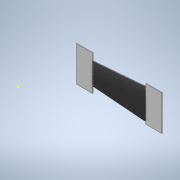
# Autodesk Inventor part: Device21
Saved by Autodesk Inventor 2020 (Build 240168000, 168)
## iProperties
Created: 2020-05-14
Part Number: Device21
Material: Generic
Document SubType Name: Modeling
Designer: nicva
Density: 1 g/cm^3
Appearance: Default
Autodesk Inventor part; units mm, degrees
ref_plane "YZ Plane" through (0, 0, 0) normal (1, 0, 0) x (0, 1, 0)
ref_plane "XZ Plane" through (0, 0, 0) normal (0, 1, 0) x (-1, 0, 0)
ref_plane "XY Plane" through (0, 0, 0) normal (0, 0, 1) x (1, 0, 0)
sketch "Sketch1" plane through (0, 0, 0) normal (0, 0, 1) x (1, 0, 0)
  point P0 (0, 0)
sketch "0" plane through (0, 0, 0) normal (0, 0, 1) x (1, 0, 0)
  line L0 (23.8209, 9.2756) -> (23.8209, 9.3229)
  line L1 (14.0209, 9.269) -> (23.8209, 9.2756)
  line L2 (14.0209, 9.303) -> (23.8209, 9.3229)
  line L3 (23.8209, 9.4649) -> (23.8209, 9.5122)
  line L4 (14.0209, 9.4049) -> (23.8209, 9.4649)
  line L5 (14.0209, 9.4389) -> (23.8209, 9.5122)
  line L6 (23.8209, 9.6542) -> (23.8209, 9.7015)
  line L7 (14.0209, 9.5409) -> (23.8209, 9.6542)
  line L8 (14.0209, 9.5749) -> (23.8209, 9.7015)
  line L9 (23.8209, 9.8435) -> (23.8209, 9.8908)
  line L10 (14.0209, 9.6769) -> (23.8209, 9.8435)
  line L11 (14.0209, 9.7109) -> (23.8209, 9.8908)
  line L12 (23.8209, 10.0328) -> (23.8209, 10.0801)
  line L13 (14.0209, 9.8129) -> (23.8209, 10.0328)
  line L14 (14.0209, 9.8469) -> (23.8209, 10.0801)
  line L15 (23.8209, 10.2221) -> (23.8209, 10.2694)
  line L16 (14.0209, 9.9489) -> (23.8209, 10.2221)
  line L17 (14.0209, 9.9829) -> (23.8209, 10.2694)
  line L18 (23.8209, 10.4113) -> (23.8209, 10.4587)
  line L19 (14.0209, 10.0848) -> (23.8209, 10.4113)
  line L20 (14.0209, 10.1188) -> (23.8209, 10.4587)
  line L21 (23.8209, 10.6006) -> (23.8209, 10.6479)
  line L22 (14.0209, 10.2208) -> (23.8209, 10.6006)
  line L23 (14.0209, 10.2548) -> (23.8209, 10.6479)
  line L24 (23.8209, 10.7899) -> (23.8209, 10.8372)
  line L25 (14.0209, 10.3568) -> (23.8209, 10.7899)
  line L26 (14.0209, 10.3908) -> (23.8209, 10.8372)
  line L27 (23.8209, 10.9792) -> (23.8209, 11.0265)
  line L28 (14.0209, 10.4928) -> (23.8209, 10.9792)
  line L29 (14.0209, 10.5268) -> (23.8209, 11.0265)
  line L30 (23.8209, 11.1685) -> (23.8209, 11.2158)
  line L31 (14.0209, 10.6288) -> (23.8209, 11.1685)
  line L32 (14.0209, 10.6628) -> (23.8209, 11.2158)
  line L33 (23.8209, 11.3578) -> (23.8209, 11.4051)
  line L34 (14.0209, 10.7648) -> (23.8209, 11.3578)
  line L35 (14.0209, 10.7988) -> (23.8209, 11.4051)
  line L36 (23.8209, 11.5471) -> (23.8209, 11.5944)
  line L37 (14.0209, 10.9007) -> (23.8209, 11.5471)
  line L38 (14.0209, 10.9347) -> (23.8209, 11.5944)
  line L39 (23.8209, 11.7363) -> (23.8209, 11.7837)
  line L40 (14.0209, 11.0367) -> (23.8209, 11.7363)
  line L41 (14.0209, 11.0707) -> (23.8209, 11.7837)
  line L42 (23.8209, 11.9256) -> (23.8209, 11.9729)
  line L43 (14.0209, 11.1727) -> (23.8209, 11.9256)
  line L44 (14.0209, 11.2067) -> (23.8209, 11.9729)
  line L45 (14.0209, 9.303) -> (14.0209, 9.4049)
  line L46 (14.0209, 9.4389) -> (14.0209, 9.5409)
  line L47 (14.0209, 9.5749) -> (14.0209, 9.6769)
  line L48 (14.0209, 9.7109) -> (14.0209, 9.8129)
  line L49 (14.0209, 9.8469) -> (14.0209, 9.9489)
  line L50 (14.0209, 9.9829) -> (14.0209, 10.0848)
  line L51 (14.0209, 10.1188) -> (14.0209, 10.2208)
  line L52 (14.0209, 10.2548) -> (14.0209, 10.3568)
  line L53 (14.0209, 10.3908) -> (14.0209, 10.4928)
  line L54 (14.0209, 10.5268) -> (14.0209, 10.6288)
  line L55 (14.0209, 10.6628) -> (14.0209, 10.7648)
  line L56 (14.0209, 10.7988) -> (14.0209, 10.9007)
  line L57 (14.0209, 10.9347) -> (14.0209, 11.0367)
  line L58 (14.0209, 11.0707) -> (14.0209, 11.1727)
  line L59 (23.8209, 9.0863) -> (23.8209, 9.1337)
  line L60 (14.0209, 9.133) -> (23.8209, 9.0863)
  line L61 (14.0209, 9.167) -> (23.8209, 9.1337)
  line L62 (23.8209, 8.8971) -> (23.8209, 8.9444)
  line L63 (14.0209, 8.997) -> (23.8209, 8.8971)
  line L64 (14.0209, 9.031) -> (23.8209, 8.9444)
  line L65 (23.8209, 8.7078) -> (23.8209, 8.7551)
  line L66 (14.0209, 8.861) -> (23.8209, 8.7078)
  line L67 (14.0209, 8.895) -> (23.8209, 8.7551)
  line L68 (23.8209, 8.5185) -> (23.8209, 8.5658)
  line L69 (14.0209, 8.725) -> (23.8209, 8.5185)
  line L70 (14.0209, 8.759) -> (23.8209, 8.5658)
  line L71 (23.8209, 8.3292) -> (23.8209, 8.3765)
  line L72 (14.0209, 8.5891) -> (23.8209, 8.3292)
  line L73 (14.0209, 8.6231) -> (23.8209, 8.3765)
  line L74 (23.8209, 8.1399) -> (23.8209, 8.1872)
  line L75 (14.0209, 8.4531) -> (23.8209, 8.1399)
  line L76 (14.0209, 8.4871) -> (23.8209, 8.1872)
  line L77 (23.8209, 7.9506) -> (23.8209, 7.9979)
  line L78 (14.0209, 8.3171) -> (23.8209, 7.9506)
  line L79 (14.0209, 8.3511) -> (23.8209, 7.9979)
  line L80 (23.8209, 7.7613) -> (23.8209, 7.8087)
  line L81 (14.0209, 8.1811) -> (23.8209, 7.7613)
  line L82 (14.0209, 8.2151) -> (23.8209, 7.8087)
  line L83 (23.8209, 7.5721) -> (23.8209, 7.6194)
  line L84 (14.0209, 8.0451) -> (23.8209, 7.5721)
  line L85 (14.0209, 8.0791) -> (23.8209, 7.6194)
  line L86 (23.8209, 7.3828) -> (23.8209, 7.4301)
  line L87 (14.0209, 7.9092) -> (23.8209, 7.3828)
  line L88 (14.0209, 7.9431) -> (23.8209, 7.4301)
  line L89 (23.8209, 7.1935) -> (23.8209, 7.2408)
  line L90 (14.0209, 7.7732) -> (23.8209, 7.1935)
  line L91 (14.0209, 7.8072) -> (23.8209, 7.2408)
  line L92 (23.8209, 7.0042) -> (23.8209, 7.0515)
  line L93 (14.0209, 7.6372) -> (23.8209, 7.0042)
  line L94 (14.0209, 7.6712) -> (23.8209, 7.0515)
  line L95 (23.8209, 6.8149) -> (23.8209, 6.8622)
  line L96 (14.0209, 7.5012) -> (23.8209, 6.8149)
  line L97 (14.0209, 7.5352) -> (23.8209, 6.8622)
  line L98 (23.8209, 6.6256) -> (23.8209, 6.6729)
  line L99 (14.0209, 7.3652) -> (23.8209, 6.6256)
  line L100 (14.0209, 7.3992) -> (23.8209, 6.6729)
  line L101 (23.8209, 6.4363) -> (23.8209, 6.4837)
  line L102 (14.0209, 7.2292) -> (23.8209, 6.4363)
  line L103 (14.0209, 7.2632) -> (23.8209, 6.4837)
  line L104 (14.0209, 9.133) -> (14.0209, 9.031)
  line L105 (14.0209, 8.997) -> (14.0209, 8.895)
  line L106 (14.0209, 8.861) -> (14.0209, 8.759)
  line L107 (14.0209, 8.725) -> (14.0209, 8.6231)
  line L108 (14.0209, 8.5891) -> (14.0209, 8.4871)
  line L109 (14.0209, 8.4531) -> (14.0209, 8.3511)
  line L110 (14.0209, 8.3171) -> (14.0209, 8.2151)
  line L111 (14.0209, 8.1811) -> (14.0209, 8.0791)
  line L112 (14.0209, 8.0451) -> (14.0209, 7.9431)
  line L113 (14.0209, 7.9092) -> (14.0209, 7.8072)
  line L114 (14.0209, 7.7732) -> (14.0209, 7.6712)
  line L115 (14.0209, 7.6372) -> (14.0209, 7.5352)
  line L116 (14.0209, 7.5012) -> (14.0209, 7.3992)
  line L117 (14.0209, 7.3652) -> (14.0209, 7.2632)
  line L118 (14.0209, 9.167) -> (14.0209, 9.269)
  line L119 (14.2209, 9.3376) -> (14.2209, 9.3719)
  line L120 (14.2209, 9.3376) -> (24.0209, 9.3709)
  line L121 (14.2209, 9.3719) -> (24.0209, 9.4185)
  line L122 (14.2209, 9.4747) -> (14.2209, 9.509)
  line L123 (14.2209, 9.4747) -> (24.0209, 9.5613)
  line L124 (14.2209, 9.509) -> (24.0209, 9.6089)
  line L125 (14.2209, 9.6118) -> (14.2209, 9.646)
  line L126 (14.2209, 9.6118) -> (24.0209, 9.7517)
  line L127 (14.2209, 9.646) -> (24.0209, 9.7993)
  line L128 (14.2209, 9.7488) -> (14.2209, 9.7831)
  line L129 (14.2209, 9.7488) -> (24.0209, 9.9421)
  line L130 (14.2209, 9.7831) -> (24.0209, 9.9897)
  line L131 (14.2209, 9.8859) -> (14.2209, 9.9202)
  line L132 (14.2209, 9.8859) -> (24.0209, 10.1324)
  line L133 (14.2209, 9.9202) -> (24.0209, 10.18)
  line L134 (14.2209, 10.023) -> (14.2209, 10.0572)
  line L135 (14.2209, 10.023) -> (24.0209, 10.3228)
  line L136 (14.2209, 10.0572) -> (24.0209, 10.3704)
  line L137 (14.2209, 10.16) -> (14.2209, 10.1943)
  line L138 (14.2209, 10.16) -> (24.0209, 10.5132)
  line L139 (14.2209, 10.1943) -> (24.0209, 10.5608)
  line L140 (14.2209, 10.2971) -> (14.2209, 10.3314)
  line L141 (14.2209, 10.2971) -> (24.0209, 10.7036)
  line L142 (14.2209, 10.3314) -> (24.0209, 10.7512)
  line L143 (14.2209, 10.4342) -> (14.2209, 10.4685)
  line L144 (14.2209, 10.4342) -> (24.0209, 10.8939)
  line L145 (14.2209, 10.4685) -> (24.0209, 10.9415)
  line L146 (14.2209, 10.5713) -> (14.2209, 10.6055)
  line L147 (14.2209, 10.5713) -> (24.0209, 11.0843)
  line L148 (14.2209, 10.6055) -> (24.0209, 11.1319)
  line L149 (14.2209, 10.7083) -> (14.2209, 10.7426)
  line L150 (14.2209, 10.7083) -> (24.0209, 11.2747)
  line L151 (14.2209, 10.7426) -> (24.0209, 11.3223)
  line L152 (14.2209, 10.8454) -> (14.2209, 10.8797)
  line L153 (14.2209, 10.8454) -> (24.0209, 11.4651)
  line L154 (14.2209, 10.8797) -> (24.0209, 11.5127)
  line L155 (14.2209, 10.9825) -> (14.2209, 11.0167)
  line L156 (14.2209, 10.9825) -> (24.0209, 11.6554)
  line L157 (14.2209, 11.0167) -> (24.0209, 11.703)
  line L158 (14.2209, 11.1195) -> (14.2209, 11.1538)
  line L159 (14.2209, 11.1195) -> (24.0209, 11.8458)
  line L160 (14.2209, 11.1538) -> (24.0209, 11.8934)
  line L161 (14.2209, 11.2566) -> (14.2209, 11.2909)
  line L162 (14.2209, 11.2566) -> (24.0209, 12.0362)
  line L163 (14.2209, 11.2909) -> (24.0209, 12.0838)
  line L164 (24.0209, 9.4185) -> (24.0209, 9.5613)
  line L165 (24.0209, 9.6089) -> (24.0209, 9.7517)
  line L166 (24.0209, 9.7993) -> (24.0209, 9.9421)
  line L167 (24.0209, 9.9897) -> (24.0209, 10.1324)
  line L168 (24.0209, 10.18) -> (24.0209, 10.3228)
  line L169 (24.0209, 10.3704) -> (24.0209, 10.5132)
  line L170 (24.0209, 10.5608) -> (24.0209, 10.7036)
  line L171 (24.0209, 10.7512) -> (24.0209, 10.8939)
  line L172 (24.0209, 10.9415) -> (24.0209, 11.0843)
  line L173 (24.0209, 11.1319) -> (24.0209, 11.2747)
  line L174 (24.0209, 11.3223) -> (24.0209, 11.4651)
  line L175 (24.0209, 11.5127) -> (24.0209, 11.6554)
  line L176 (24.0209, 11.703) -> (24.0209, 11.8458)
  line L177 (24.0209, 11.8934) -> (24.0209, 12.0362)
  line L178 (14.2209, 9.2006) -> (14.2209, 9.2348)
  line L179 (14.2209, 9.2006) -> (24.0209, 9.1806)
  line L180 (14.2209, 9.2348) -> (24.0209, 9.2282)
  line L181 (14.2209, 9.0635) -> (14.2209, 9.0978)
  line L182 (14.2209, 9.0635) -> (24.0209, 8.9902)
  line L183 (14.2209, 9.0978) -> (24.0209, 9.0378)
  line L184 (14.2209, 8.9264) -> (14.2209, 8.9607)
  line L185 (14.2209, 8.9264) -> (24.0209, 8.7998)
  line L186 (14.2209, 8.9607) -> (24.0209, 8.8474)
  line L187 (14.2209, 8.7894) -> (14.2209, 8.8236)
  line L188 (14.2209, 8.7894) -> (24.0209, 8.6095)
  line L189 (14.2209, 8.8236) -> (24.0209, 8.657)
  line L190 (14.2209, 8.6523) -> (14.2209, 8.6866)
  line L191 (14.2209, 8.6523) -> (24.0209, 8.4191)
  line L192 (14.2209, 8.6866) -> (24.0209, 8.4667)
  line L193 (14.2209, 8.5152) -> (14.2209, 8.5495)
  line L194 (14.2209, 8.5152) -> (24.0209, 8.2287)
  line L195 (14.2209, 8.5495) -> (24.0209, 8.2763)
  line L196 (14.2209, 8.3782) -> (14.2209, 8.4124)
  line L197 (14.2209, 8.3782) -> (24.0209, 8.0383)
  line L198 (14.2209, 8.4124) -> (24.0209, 8.0859)
  line L199 (14.2209, 8.2411) -> (14.2209, 8.2753)
  line L200 (14.2209, 8.2411) -> (24.0209, 7.848)
  line L201 (14.2209, 8.2753) -> (24.0209, 7.8956)
  line L202 (14.2209, 8.104) -> (14.2209, 8.1383)
  line L203 (14.2209, 8.104) -> (24.0209, 7.6576)
  line L204 (14.2209, 8.1383) -> (24.0209, 7.7052)
  line L205 (14.2209, 7.9669) -> (14.2209, 8.0012)
  line L206 (14.2209, 7.9669) -> (24.0209, 7.4672)
  line L207 (14.2209, 8.0012) -> (24.0209, 7.5148)
  line L208 (14.2209, 7.8299) -> (14.2209, 7.8641)
  line L209 (14.2209, 7.8299) -> (24.0209, 7.2768)
  line L210 (14.2209, 7.8641) -> (24.0209, 7.3244)
  line L211 (14.2209, 7.6928) -> (14.2209, 7.7271)
  line L212 (14.2209, 7.6928) -> (24.0209, 7.0865)
  line L213 (14.2209, 7.7271) -> (24.0209, 7.1341)
  line L214 (14.2209, 7.5557) -> (14.2209, 7.59)
  line L215 (14.2209, 7.5557) -> (24.0209, 6.8961)
  line L216 (14.2209, 7.59) -> (24.0209, 6.9437)
  line L217 (14.2209, 7.4187) -> (14.2209, 7.4529)
  line L218 (14.2209, 7.4187) -> (24.0209, 6.7057)
  line L219 (14.2209, 7.4529) -> (24.0209, 6.7533)
  line L220 (14.2209, 7.2816) -> (14.2209, 7.3159)
  line L221 (14.2209, 7.2816) -> (24.0209, 6.5153)
  line L222 (14.2209, 7.3159) -> (24.0209, 6.5629)
  line L223 (24.0209, 9.1806) -> (24.0209, 9.0378)
  line L224 (24.0209, 8.9902) -> (24.0209, 8.8474)
  line L225 (24.0209, 8.7998) -> (24.0209, 8.657)
  line L226 (24.0209, 8.6095) -> (24.0209, 8.4667)
  line L227 (24.0209, 8.4191) -> (24.0209, 8.2763)
  line L228 (24.0209, 8.2287) -> (24.0209, 8.0859)
  line L229 (24.0209, 8.0383) -> (24.0209, 7.8956)
  line L230 (24.0209, 7.848) -> (24.0209, 7.7052)
  line L231 (24.0209, 7.6576) -> (24.0209, 7.5148)
  line L232 (24.0209, 7.4672) -> (24.0209, 7.3244)
  line L233 (24.0209, 7.2768) -> (24.0209, 7.1341)
  line L234 (24.0209, 7.0865) -> (24.0209, 6.9437)
  line L235 (24.0209, 6.8961) -> (24.0209, 6.7533)
  line L236 (24.0209, 6.7057) -> (24.0209, 6.5629)
  line L237 (24.0209, 9.2282) -> (24.0209, 9.3709)
  line L238 (24.0209, 6.5153) -> (24.0209, 6.0153)
  line L239 (24.0209, 12.0838) -> (24.0209, 12.5838)
  line L240 (24.0209, 6.0153) -> (27.0209, 6.0153)
  line L241 (24.0209, 12.5838) -> (27.0209, 12.5838)
  line L242 (27.0209, 6.0153) -> (27.0209, 12.5838)
  line L243 (14.0209, 7.2292) -> (14.0209, 6.0153)
  line L244 (14.0209, 11.2067) -> (14.0209, 12.5838)
  line L245 (14.0209, 6.0153) -> (11.0209, 6.0153)
  line L246 (14.0209, 12.5838) -> (11.0209, 12.5838)
  line L247 (11.0209, 6.0153) -> (11.0209, 12.5838)
  constraints: 496 end point
extrude "Extrusion1" add sketch "0" along normal blind 0.127
body "Solid1"
